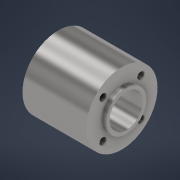
# Autodesk Inventor part: shaft
Saved by Autodesk Inventor 2021.3 (Build 253353000, 353)
## iProperties
Created: 2021-10-17
Part Number: shaft
Material: Stainless Steel
Document SubType Name: Modeling
Designer: ASUS
Density: 8 g/cm^3
Appearance: Semi-Polished
Author: ASUS
Autodesk Inventor part; units mm, degrees
ref_plane "YZ Plane" through (0, 0, 0) normal (1, 0, 0) x (0, 1, 0)
ref_plane "XZ Plane" through (0, 0, 0) normal (0, 1, 0) x (-1, 0, 0)
ref_plane "XY Plane" through (0, 0, 0) normal (0, 0, 1) x (1, 0, 0)
sketch "Sketch1" plane through (0, 0, 0) normal (0, 1, 0) x (-1, 0, 0)
  line L0 (14.234, 0) -> (-14.234, 0)
  line L1 (14.234, 0) -> (14.234, -16)
  line L2 (14.234, -16) -> (-14.234, -16)
  line L3 (-14.234, 0) -> (-14.234, -16)
  line L4 (16.234, 0) -> (16.234, -8.975)
  line L5 (16.234, -8.975) -> (14.234, -8.975)
  line L6 (16.234, 0) -> (14.234, 0)
  line L7 (0, 0) -> (0, -16) construction
  line L8 (-16.234, 0) -> (-16.234, -8.975)
  line L9 (-16.234, -8.975) -> (-14.234, -8.975)
  line L10 (-16.234, 0) -> (-14.234, 0)
  point P0 (-14.234, -8.975)
  dimension "d0" = 28.468
  dimension "d1" = 16
  dimension "d2" = 8.975
  dimension "d3" = 2
  dimension "d52" = 16
  dimension "d53" = 14.234
  dimension "d54" = 14.234
  dimension "d55" = 32.468
  constraints: 22 end point, 3 perpendicular, 3 symmetric about line, 2 vertical, 1 horizontal, 1 midpoint, 1 parallel, 1 point on line
  measures "d0" distance of L0.start L0.end
  measures "d1" distance of L0.start L1.end
  measures "d2" distance of L4.start L4.end
  measures "d3" distance between parallel lines of L1 L4
  measures "d52" distance of L7.start L7.end
  measures "d53" distance of L0.end L7.start
  measures "d54" distance of L0.start L7.start
  measures "d55" distance of L8.start L4.start
revolve "Revolution1" add sketch "Sketch1" angle 360 about axis through (-14.234, 0, 0) along (1, 0, 0)
sketch "Sketch3" plane through (14.234, 0, 0) normal (1, 0, 0) x (0, 0, -1)
  line L0 (0, 0) -> (0, 21.0687)
  circle A0 centre (0, 0) radius 12
  line L1 (0, 0) -> (15.1968, 15.1968)
  circle A1 centre (8.4853, 8.4853) radius 1.5075
  dimension "d12" = 24
  dimension "d13" = 45
  dimension "d14" = 3.015
  constraints: 4 end point, 1 centre point, 1 coincident, 1 point on line, 1 vertical, 3 other
  measures "d13" angle of L1 L0
  measures "d14" diameter of A1
extrude "Extrusion1" cut sketch "Sketch3" against normal through all contours A1 A0 L1 | L1 A0 A1 | A1 L1 A0 | L1 A1 A0
thread "Thread1" size "M3x0.5" class "6H" standard "ANSI Metric M Profile" full length
sketch "Sketch5" plane through (16.234, 0, 0) normal (1, 0, 0) x (0, 0, -1)
  circle A0 centre (0, 0) radius 8.975 projected
  point P0 (0, 0)
  constraints: 1 coincident
hole "Hole3" at (16.234, 0, 0) direction (-1, 0, 0) diameter 15 end through all
pattern_circular "Circular Pattern3" count 4 over 360 about axis through (-39.4631, 0, 0) along (1, 0, 0) of "Extrusion1"
body "Solid1"
